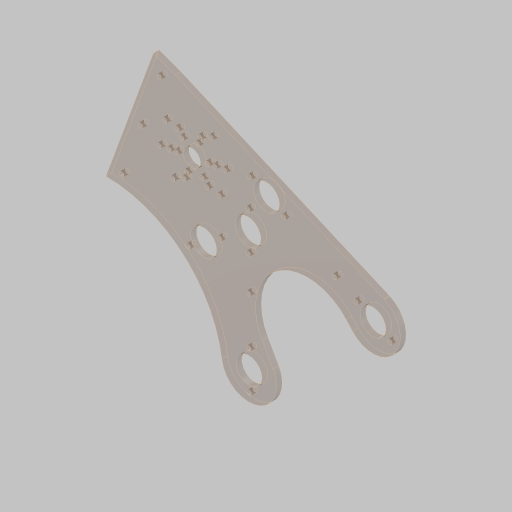
# Autodesk Inventor part: GP7-001
Saved by Autodesk Inventor 2023.5 (Build 275446000, 446)
## iProperties
Created: 2025-02-24
Part Number: GP7-001
Material: Polycarbonate, Smoke
Document SubType Name: Modeling
Designer: dlangdon
Density: 1.2 g/cm^3
Appearance: Polycarbonate - Smoked
Author: dlangdon
Autodesk Inventor part; units mm, degrees
ref_plane "YZ Plane" through (0, 0, 0) normal (1, 0, 0) x (0, 1, 0)
ref_plane "XZ Plane" through (0, 0, 0) normal (0, 1, 0) x (-1, 0, 0)
ref_plane "XY Plane" through (0, 0, 0) normal (0, 0, 1) x (1, 0, 0)
sketch "Sketch1" plane through (0, 0, 0) normal (0, 0, 1) x (1, 0, 0)
  circle A0 centre (68.1014, 57.1438) radius 38.1 construction
  circle A1 centre (-68.1014, -57.1438) radius 38.1 construction
  circle A2 centre (0, 0) radius 50.8 construction
  line L0 (-38.9151, -32.6536) -> (38.9151, 32.6536) construction
  line L1 (68.1014, 57.1438) -> (-68.1014, -57.1438) construction
  line L2 (-3.81, 6.5991) -> (-3.81, 50.6569) construction
  line L3 (-399.8199, -95.2438) -> (465.5721, -95.2438) construction
  circle A3 centre (151.5813, -38.0938) radius 57.15 construction
  circle A4 centre (68.1014, 57.1438) radius 14.2621
  circle A5 centre (-68.1014, -57.1438) radius 14.2621
  circle A6 centre (-3.81, 6.5991) radius 57.15 construction
  circle A7 centre (-68.1014, -57.1438) radius 30.1371 construction
  circle A8 centre (68.1014, 57.1438) radius 30.1371 construction
  circle A9 centre (-48.8413, 117.4952) radius 14.2621
  line L4 (-48.8413, 117.4952) -> (68.1014, 57.1438) construction
  circle A10 centre (68.1014, 57.1438) radius 14.2875 construction
  circle A11 centre (-68.1014, -57.1438) radius 14.2875 construction
  circle A12 centre (-69.3038, 74.4481) radius 14.2621
  line L5 (-68.1014, -57.1438) -> (-69.3038, 74.4481) construction
  circle A13 centre (-69.3038, 74.4481) radius 23.8316 construction
  circle A14 centre (-48.8413, 117.4952) radius 23.8316 construction
  line L6 (38.7541, 44.736) -> (45.6559, 37.033)
  line L7 (-41.8356, -42.367) -> (-53.6186, -21.4227)
  arc A15 (38.7541, 44.736) -> (-53.6186, -21.4227) centre (-3.81, 6.5991) ccw
  line L8 (-173.2789, 192.3018) -> (-149.4107, 183.6144)
  line L9 (-149.4107, 183.6144) -> (-201.5346, 40.4053) construction
  line L10 (-201.5346, 40.4053) -> (-225.4028, 49.0926) construction
  line L11 (-225.4028, 49.0926) -> (-173.2789, 192.3018) construction
  line L12 (-254.1767, -29.9631) -> (29.2993, -133.1399) construction
  line L13 (-175.4508, 186.3347) -> (194.0315, 51.8542) construction
  line L14 (-175.4508, 186.3347) -> (-254.1767, -29.9631) construction
  circle A16 centre (-130.9364, 113.6923) radius 31.75 construction
  line L15 (-69.086, 50.6175) -> (-68.4495, -19.0454) construction
  circle A17 centre (25.7799, 78.985) radius 9.525 construction
  line L16 (-161.3448, 187.9581) -> (-213.4687, 44.7489) construction
  line L17 (-166.7744, 173.0405) -> (-208.0391, 59.6666) construction
  circle A18 centre (-130.9364, 113.6923) radius 17.4625 construction
  circle A19 centre (-130.9364, 113.6923) radius 9.525
  circle A20 centre (-48.8413, 117.4952) radius 30.1816 construction
  line L18 (-173.2789, 192.3018) -> (-225.4028, 49.0926)
  arc A21 (45.6559, 37.033) -> (80.0201, 84.8239) centre (68.1014, 57.1438) ccw
  arc A22 (-97.9473, -61.3229) -> (-41.8356, -42.367) centre (-68.1014, -57.1438) ccw
  line L19 (-130.9364, 113.6923) -> (-113.7392, 116.7246) construction
  line L20 (-94.9786, 120.0326) -> (-166.8942, 107.3519) construction
  circle A23 centre (-166.8942, 107.3519) radius 4.7625 construction
  line L21 (0, 0) -> (-3.81, 6.5991) construction
  circle A24 centre (68.1014, 57.1438) radius 28.6512 construction
  line L22 (52.2566, 33.2726) -> (-56.7285, 105.6125) construction
  line L23 (78.3783, 83.8885) -> (-43.7256, 130.8083) construction
  line L24 (-149.4107, 183.6144) -> (80.0201, 84.8239)
  line L25 (-130.9364, 113.6923) -> (-117.8841, 39.766) construction
  circle A25 centre (-117.8841, 39.766) radius 31.75 construction
  circle A26 centre (-117.8841, 39.766) radius 14.2621
  line L26 (-69.3038, 74.4481) -> (-117.8841, 39.766) construction
  circle A27 centre (-130.9364, 113.6923) radius 25.4 construction
  arc A28 (-97.9473, -61.3229) -> (-225.4028, 49.0926) centre (-224.9018, -79.0994) ccw
  circle A29 centre (-130.9364, 113.6923) radius 36.5125 construction
  line L27 (-160.8457, 134.635) -> (-130.9364, 113.6923) construction
  point P0 (-68.7678, 15.7861)
  point P1 (-187.4068, 116.3535)
  point P2 (-187.4068, 116.3535)
  point P3 (-124.9639, 130.1017)
  point P4 (-142.1611, 127.0693)
  point P5 (-148.1336, 110.6599)
  point P6 (-136.9089, 97.2829)
  point P7 (-119.7117, 100.3152)
  point P8 (-105.9223, 118.1029)
  point P9 (-122.2491, 137.5605)
  point P10 (-147.2632, 133.1498)
  point P11 (-155.9505, 109.2816)
  point P12 (-139.6237, 89.8241)
  point P13 (-114.6096, 94.2347)
  point P14 (-137.2767, 149.6501)
  point P15 (-166.8942, 107.3519)
  point P16 (-124.5961, 77.7345)
  point P17 (-109.9937, 143.6016)
  point P18 (-151.8791, 83.783)
  point P19 (-101.0271, 92.7496)
  dimension "d7" = 76.2
  dimension "d18" = 47.6631
  dimension "d34" = 34.925
  dimension "d65" = 50.8
  dimension "d3" = 50
  dimension "d4" = 0
  dimension "d8" = 101.6
  dimension "d9" = 28.5242
  dimension "d10" = 76.2
  dimension "d11" = 114.3
  dimension "d12" = 114.3
  dimension "d13" = 15.875
  dimension "d14" = 15.875
  dimension "d15" = 131.5974
  dimension "d16" = 28.575
  dimension "d17" = 131.5974
  dimension "d19" = 47.6631
  dimension "d22" = 25.4
  dimension "d23" = 152.4
  dimension "d26" = 230.1793
  dimension "d27" = 63.5
  dimension "d30" = 203.2
  dimension "d31" = 20
  dimension "d32" = 19.05
  dimension "d33" = 120.65
  dimension "d35" = 19.05
  dimension "d36" = 6.35
  dimension "d40" = 360
  dimension "d44" = 9.525
  dimension "d55" = 80
  dimension "d56" = 7.62
  dimension "d58" = 57.3024
  dimension "d59" = 63.5
  dimension "d60" = 75.0697
  dimension "d61" = 59.69
  dimension "d62" = 55
  dimension "d68" = 360
  dimension "d70" = 41.275
  dimension "d71" = 60
  dimension "d82" = 360
  dimension "d87" = 360
  dimension "d89" = 45
  dimension "d90" = 6.35
  dimension "d91" = 20.955
  constraints: 56 end point, 26 centre point, 24 coincident, 23 point on circle, 16 tangent, 7 midpoint, 5 equal radius, 5 point on line, 4 collinear, 4 parallel, 2 horizontal, 1 concentric, 1 perpendicular, 1 vertical, 39 other
  measures "d3" angle of L2 L0
  measures "d4" distance between parallel lines of L0 L1
  measures "d8" diameter of A2
  measures "d9" diameter of A4
  measures "d10" diameter of A0
  measures "d11" diameter of A3
  measures "d12" diameter of A6
  measures "d13" radial gap between concentric circles of A5 A7
  measures "d14" radial gap between concentric circles of A4 A8
  measures "d15" distance of L4.start L4.end
  measures "d16" diameter of A10
  measures "d17" distance of L5.start L5.end
  measures "d19" diameter of A14
  measures "d22" distance of L9.end L10.end
  measures "d23" distance of L10.end L8.start
  measures "d26" distance of L13.start L12.start
  measures "d27" diameter of A16
  measures "d30" distance from line of point (0, 0) L9
  measures "d31" angle of L3 L12
  measures "d32" diameter of A17
  measures "d33" distance of L17.start L17.end
  measures "d35" diameter of A19
  measures "d36" radial gap between concentric circles of A14 A20
  measures "d44" diameter of A23
  measures "d55" angle of L1 L21
  measures "d56" distance of L21.start L21.end
  measures "d58" diameter of A24
  measures "d59" diameter of A25
  measures "d60" distance of L19.start L25.end
  measures "d61" distance of L26.start L26.end
  measures "d62" angle of L15 L26
  measures "d70" distance from line of L9 L19.start
  measures "d71" angle of L9 L20
  measures "d89" angle of L20 L27
  measures "d90" distance between parallel lines of L8 L13
  measures "d91" distance from line of L24 L4.start
extrude "Extrusion1" add sketch "Sketch1" along normal blind 6.35
hole "Hole1" at (25.7799, 78.985, 0) at (-166.7744, 173.0405, 0) at (-187.4068, 116.3535, 0) at (-208.0391, 59.6666, 0) at (-113.7392, 116.7246, 0) at (-124.9639, 130.1017, 0) at (-142.1611, 127.0693, 0) at (-148.1336, 110.6599, 0) at (-136.9089, 97.2829, 0) at (-119.7117, 100.3152, 0) at (-94.9786, 120.0326, 0) at (-166.8942, 107.3519, 0) at (-139.6237, 89.8241, 0) at (-155.9505, 109.2816, 0) at (-147.2632, 133.1498, 0) at (-122.2491, 137.5605, 0) at (-105.9223, 118.1029, 0) at (-114.6096, 94.2347, 0) at (-68.7678, 15.7861, 0) at (-160.8457, 134.635, 0) at (-109.9937, 143.6016, 0) at (-101.0271, 92.7496, 0) at (-151.8791, 83.783, 0) direction (0, 0, 1) diameter 5.1054 end through all clearance for "Flat Head Machine Screw (82)" size "#10" standard "Ansi Unified Screw Threads"
sketch "Sketch2" plane through (0, 0, 6.35) normal (0, 0, 1) x (1, 0, 0)
  circle A0 centre (-114.6096, 94.2347) radius 2.5527 construction
  circle A1 centre (-122.2491, 137.5605) radius 2.5527 construction
  circle A2 centre (-155.9505, 109.2816) radius 2.5527 construction
  circle A3 centre (-166.8942, 107.3519) radius 2.5527 construction
  circle A4 centre (-119.7117, 100.3152) radius 2.5527 construction
  circle A5 centre (-148.1336, 110.6599) radius 2.5527 construction
  circle A6 centre (-124.9639, 130.1017) radius 2.5527 construction
  circle A7 centre (-208.0391, 59.6666) radius 2.5527 construction
  circle A8 centre (-166.7744, 173.0405) radius 2.5527 construction
  circle A9 centre (25.7799, 78.985) radius 2.5527 construction
  circle A10 centre (-187.4068, 116.3535) radius 2.5527 construction
  circle A11 centre (-113.7392, 116.7246) radius 2.5527 construction
  circle A12 centre (-142.1611, 127.0693) radius 2.5527 construction
  circle A13 centre (-136.9089, 97.2829) radius 2.5527 construction
  circle A14 centre (-94.9786, 120.0326) radius 2.5527 construction
  circle A15 centre (-139.6237, 89.8241) radius 2.5527 construction
  circle A16 centre (-147.2632, 133.1498) radius 2.5527 construction
  circle A17 centre (-105.9223, 118.1029) radius 2.5527 construction
  circle A18 centre (-68.7678, 15.7861) radius 2.5527 construction
  line L0 (-41.8356, -42.367) -> (-53.6186, -21.4227) construction
  arc A19 (38.7541, 44.736) -> (-53.6186, -21.4227) centre (-3.81, 6.5991) ccw construction
  line L1 (38.7541, 44.736) -> (45.6559, 37.033) construction
  arc A20 (45.6559, 37.033) -> (80.0201, 84.8239) centre (68.1014, 57.1438) ccw construction
  line L2 (80.0201, 84.8239) -> (-149.4107, 183.6144) construction
  line L3 (-149.4107, 183.6144) -> (-173.2789, 192.3018) construction
  line L4 (-173.2789, 192.3018) -> (-225.4028, 49.0926) construction
  arc A21 (-97.9473, -61.3229) -> (-225.4028, 49.0926) centre (-224.9018, -79.0994) ccw construction
  arc A22 (-97.9473, -61.3229) -> (-41.8356, -42.367) centre (-68.1014, -57.1438) ccw construction
  circle A23 centre (-69.3038, 74.4481) radius 14.2621 construction
  circle A24 centre (-130.9364, 113.6923) radius 9.525 construction
  circle A25 centre (-117.8841, 39.766) radius 14.2621 construction
  circle A26 centre (-48.8413, 117.4952) radius 14.2621 construction
  circle A27 centre (-68.1014, -57.1438) radius 14.2621 construction
  circle A28 centre (68.1014, 57.1438) radius 14.2621 construction
  line L5 (-68.2934, -36.1262) -> (-67.9093, -78.1614) construction
  line L6 (-134.9906, 27.5534) -> (-100.7776, 51.9785) construction
  line L7 (-69.4958, 95.4657) -> (-69.1117, 53.4305) construction
  line L8 (-67.5192, 127.1345) -> (-30.1634, 107.856) construction
  line L9 (49.4235, 66.783) -> (86.7792, 47.5046) construction
  circle A29 centre (-69.3038, 74.4481) radius 14.2621 construction
  line L10 (-48.8413, 117.4952) -> (-69.3038, 74.4481) construction
  line L11 (-48.8413, 117.4952) -> (68.1014, 57.1438) construction
  line L12 (-69.3038, 74.4481) -> (-117.8841, 39.766) construction
  line L13 (-69.3038, 74.4481) -> (-68.1014, -57.1438) construction
  circle A30 centre (-101.0271, 92.7496) radius 2.5527 projected
  point P0 (0, 0)
  point P1 (-116.0598, 70.5176)
  point P2 (-113.1961, 73.3575)
  dimension "d72" = 42.037
  constraints: 19 end point, 14 coincident, 5 collinear, 5 midpoint, 4 equal length, 1 other
  measures "d72" distance of L5.start L5.end
hole "Hole2" at (-68.2934, -36.1262, 6.35) at (-100.7776, 51.9785, 6.35) at (-67.9093, -78.1614, 6.35) at (-134.9906, 27.5534, 6.35) at (-69.1117, 53.4305, 6.35) at (-69.4958, 95.4657, 6.35) at (-30.1634, 107.856, 6.35) at (-67.5192, 127.1345, 6.35) at (86.7792, 47.5046, 6.35) at (49.4235, 66.783, 6.35) direction (0, 0, -1) diameter 5.1054 end through all clearance for "Flat Head Machine Screw (82)" size "#10" standard "Ansi Unified Screw Threads"
body "Solid1"
